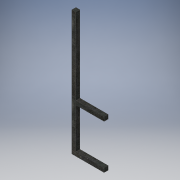
# Autodesk Inventor part: support
Saved by Autodesk Inventor 2019 (Build 230136000, 136)
## iProperties
Created: 2021-03-08
Part Number: support
Material: Steel
Document SubType Name: Modeling
Designer: User
Density: 7.85 g/cm^3
Appearance: Plate
Author: User
Autodesk Inventor part; units mm, degrees
ref_plane "YZ Plane" through (0, 0, 0) normal (1, 0, 0) x (0, 1, 0)
ref_plane "XZ Plane" through (0, 0, 0) normal (0, 1, 0) x (-1, 0, 0)
ref_plane "XY Plane" through (0, 0, 0) normal (0, 0, 1) x (1, 0, 0)
sketch "Sketch2" plane through (0, 0, 0) normal (0, 0, 1) x (1, 0, 0)
  line L0 (0, 310) -> (0, 0)
  line L1 (0, 0) -> (10, 0)
  line L2 (10, 0) -> (10, 0)
  line L3 (10, 0) -> (80, 0)
  line L4 (80, 0) -> (80, 10)
  line L5 (80, 10) -> (10, 10)
  line L6 (10, 10) -> (10, 110)
  line L7 (10, 110) -> (80, 110)
  line L8 (80, 110) -> (80, 120)
  line L9 (80, 120) -> (10, 120)
  line L10 (10, 120) -> (10, 310)
  line L11 (10, 310) -> (0, 310)
  dimension "d12" = 100
  dimension "d13" = 10
  dimension "d14" = 10
  dimension "d15" = 10
  dimension "d16" = 10
  dimension "d17" = 190
  dimension "d18" = 310
  dimension "d19" = 80
  constraints: 24 end point, 8 perpendicular, 3 point on line, 2 vertical
  measures "d12" distance between parallel lines of L5 L7
  measures "d13" distance between parallel lines of L2 L0
  measures "d14" distance between parallel lines of L3 L5
  measures "d15" distance between parallel lines of L7 L9
  measures "d16" distance between parallel lines of L0 L10
  measures "d17" distance between parallel lines of L9 L11
  measures "d18" distance between parallel lines of L1 L11
  measures "d19" distance from line of L7.end L0
extrude "Extrusion2" add sketch "Sketch2" along normal mid plane 10
body "Solid2"
